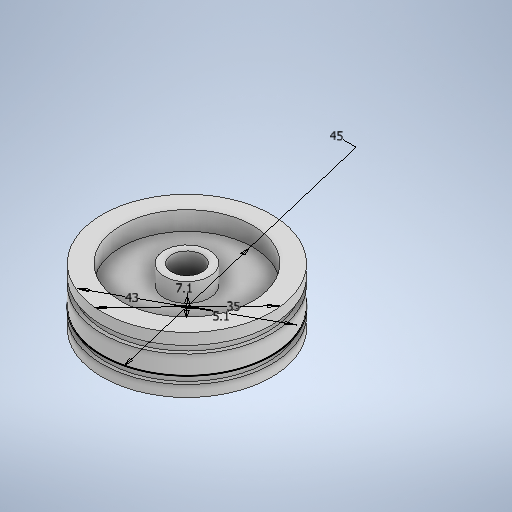
# Autodesk Inventor part: roller
Saved by Autodesk Inventor 2025.1 (Build 291241020, 241B)
## iProperties
Created: 2025-01-25
Part Number: roller
Material: Generic
Document SubType Name: Modeling
Designer: User
Density: 1 g/cm^3
Appearance: Default
Author: User
Autodesk Inventor part; units mm, degrees
ref_plane "YZ Plane" through (0, 0, 0) normal (1, 0, 0) x (0, 1, 0)
ref_plane "XZ Plane" through (0, 0, 0) normal (0, 1, 0) x (-1, 0, 0)
ref_plane "XY Plane" through (0, 0, 0) normal (0, 0, 1) x (1, 0, 0)
sketch "Sketch1" plane through (0, 0, 0) normal (0, 1, 0) x (-1, 0, 0)
  circle A0 centre (0, 0) radius 22.5
  circle A1 centre (0, 0) radius 2.55
  circle A2 centre (0, 0) radius 17.5
  circle A3 centre (0, 0) radius 21.5
  circle A4 centre (0, 0) radius 3.55
  dimension "d0" = 45
  dimension "d1" = 5.1
  dimension "d2" = 35
  dimension "d9" = 43
  dimension "d16" = 7.1
  constraints: 5 centre point, 5 coincident
  measures "d0" diameter of A0
  measures "d1" diameter of A1
  measures "d2" diameter of A2
  measures "d9" diameter of A3
  measures "d16" diameter of A4
extrude "Extrusion1" add sketch "Sketch1" along normal blind 5 contours A2 | A4
extrude "Extrusion2" add sketch "Sketch1" along normal blind 10 contours A0 | A3
extrude "Extrusion3" add sketch "Sketch1" against normal blind 5 contours A0 | A3
extrude "Extrusion4" cut sketch "Sketch1" against normal blind 2 contours A0
sketch "Sketch2" plane through (0, 5, 0) normal (0, 1, 0) x (1, 0, 0)
  circle A0 centre (0, 0) radius 22.5
  circle A1 centre (0, 0) radius 21.5
  dimension "d12" = 45
  dimension "d13" = 43
  constraints: 2 centre point, 2 coincident
  measures "d12" diameter of A0
  measures "d13" diameter of A1
extrude "Extrusion5" cut sketch "Sketch2" along normal blind 2
extrude "Extrusion6" add sketch "Sketch1" against normal blind 5 contours A4
extrude "Extrusion7" add sketch "Sketch1" along normal blind 10 contours A4
sketch "Sketch3" plane through (0, 10, 0) normal (0, 1, 0) x (1, 0, 0)
  circle A0 centre (0, 0) radius 4.05
  circle A1 centre (0, 0) radius 6
  dimension "d21" = 8.1
  dimension "d22" = 12
  constraints: 2 centre point, 2 coincident
  measures "d21" diameter of A0
  measures "d22" diameter of A1
extrude "Extrusion8" add sketch "Sketch3" against normal blind 15
extrude "Extrusion9" cut sketch "Sketch3" against normal through all contours A0
body "Solid1"
